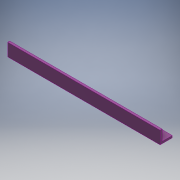
# Autodesk Inventor part: repisa
Saved by Autodesk Inventor 2018 (Build 220112000, 112)
## iProperties
Created: 2018-01-24
Part Number: repisa
Material: Generic
Document SubType Name: Modeling
Designer: mokuz
Density: 1 g/cm^3
Appearance: Smooth - Purple
Author: mokuz
Autodesk Inventor part; units mm, degrees
ref_plane "YZ Plane" through (0, 0, 0) normal (1, 0, 0) x (0, 1, 0)
ref_plane "XZ Plane" through (0, 0, 0) normal (0, 1, 0) x (-1, 0, 0)
ref_plane "XY Plane" through (0, 0, 0) normal (0, 0, 1) x (1, 0, 0)
sketch "Sketch1" plane through (0, 0, 0) normal (0, 0, 1) x (1, 0, 0)
  line L0 (0, 0) -> (1200, 0)
  line L1 (1200, 0) -> (1200, 16)
  line L2 (1200, 16) -> (0, 16)
  line L3 (0, 16) -> (0, 0)
  dimension "d0" = 1200
  dimension "d1" = 16
  constraints: 8 end point, 2 perpendicular, 1 horizontal, 1 parallel
  measures "d0" distance of L0.start L0.end
  measures "d1" distance of L0.end L1.end
extrude "Extrusion1" add sketch "Sketch1" along normal blind 100
sketch "Sketch2" plane through (0, 16, 0) normal (0, 1, 0) x (1, 0, 0)
  line L0 (1200, 0) -> (0, 0) projected
  line L1 (0, 0) -> (0, -100) projected
  line L2 (1200, -100) -> (0, -100) projected
  line L3 (1200, 0) -> (1200, -100) projected
  line L4 (0, 0) -> (0, -100) projected
  line L5 (1200, 0) -> (0, 0)
  line L6 (0, 0) -> (0, -16)
  line L7 (0, -16) -> (1200, -16)
  line L8 (1200, -16) -> (1200, 0)
  dimension "d4" = 16
  constraints: 8 end point, 2 parallel, 1 horizontal, 1 perpendicular, 1 point on line
  measures "d4" distance of L6.end L5.end
extrude "Extrusion2" add sketch "Sketch2" along normal blind 80 contours L3 L7 L1 L0
body "Solid1"
